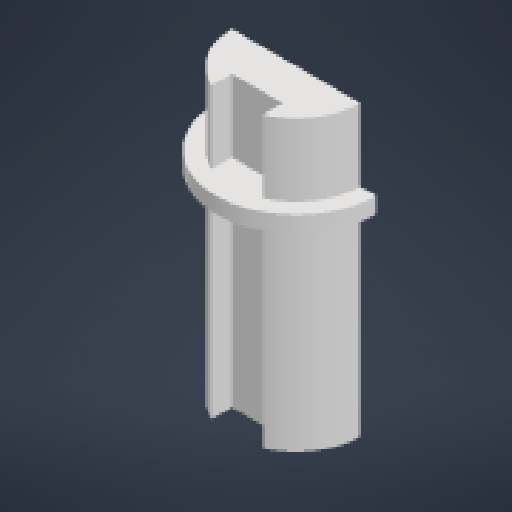
# Autodesk Inventor part: halfAxel
Saved by Autodesk Inventor 2026 (Build 300175050, 175E)
## iProperties
Created: 2026-04-30
Part Number: halfAxel
Material: Generic
Document SubType Name: Modeling
Designer: sniel
Density: 1 g/cm^3
Appearance: Default
Author: sniel
Autodesk Inventor part; units mm, degrees
ref_plane "YZ Plane" through (0, 0, 0) normal (1, 0, 0) x (0, 1, 0)
ref_plane "XZ Plane" through (0, 0, 0) normal (0, 1, 0) x (-1, 0, 0)
ref_plane "XY Plane" through (0, 0, 0) normal (0, 0, 1) x (1, 0, 0)
sketch "Sketch1" plane through (0, 0, 0) normal (0, 1, 0) x (-1, 0, 0)
  circle A0 centre (0, 0) radius 4
  line L0 (-1.575, 5.575) -> (1.575, 5.575)
  line L1 (1.575, 5.575) -> (1.575, 2.425)
  line L2 (1.575, 2.425) -> (-1.575, 2.425)
  line L3 (-1.575, 2.425) -> (-1.575, 5.575)
  line L4 (-1.575, 5.575) -> (1.575, 2.425) construction
  line L5 (1.575, 5.575) -> (-1.575, 2.425) construction
  line L6 (-1.575, -2.425) -> (1.575, -2.425)
  line L7 (1.575, -2.425) -> (1.575, -5.575)
  line L8 (1.575, -5.575) -> (-1.575, -5.575)
  line L9 (-1.575, -5.575) -> (-1.575, -2.425)
  line L10 (-1.575, -2.425) -> (1.575, -5.575) construction
  line L11 (1.575, -2.425) -> (-1.575, -5.575) construction
  point P0 (0, 0)
  point P1 (0, 4)
  point P2 (0, -4)
  point P3 (-1.575, 3.6769)
  point P4 (-1.575, -3.6769)
  point P5 (1.575, -3.6769)
  point P6 (1.575, 3.6769)
  dimension "d0" = 8
  dimension "d10" = 3.15
  dimension "d11" = 3.15
  dimension "d12" = 3.15
  dimension "d13" = 3.15
  constraints: 24 end point, 4 midpoint, 4 parallel, 2 horizontal, 2 perpendicular, 2 point on circle, 1 centre point
  measures "d0" diameter of A0
  measures "d10" distance of L1.end L2.end
  measures "d11" distance of L0.end L1.end
  measures "d12" distance of L7.end L8.end
  measures "d13" distance of L6.end L7.end
extrude "Extrusion1" add sketch "Sketch1" along normal blind 5 and the other way blind 13 contours A0 L7 L6 L9 L3 L2 L1
sketch "Sketch2" plane through (0, 0, 0) normal (0, 1, 0) x (-1, 0, 0)
  circle A0 centre (0, 0) radius 5
  dimension "d3" = 10
  constraints: 1 centre point, 1 coincident
  measures "d3" diameter of A0
extrude "Extrusion2" add sketch "Sketch2" along normal mid plane 1
sketch "Sketch3" plane through (0, 5, 0) normal (0, 1, 0) x (0, 0, 1)
  line L0 (0, -14) -> (-10, -14)
  line L1 (-10, -14) -> (-10, 12)
  line L2 (-10, 12) -> (0, 12)
  line L3 (0, 12) -> (0, -14)
  point P0 (0, 0)
  constraints: 8 end point, 2 parallel, 1 horizontal, 1 perpendicular
extrude "Extrusion3" cut sketch "Sketch3" against normal blind 22
body "Solid1"
